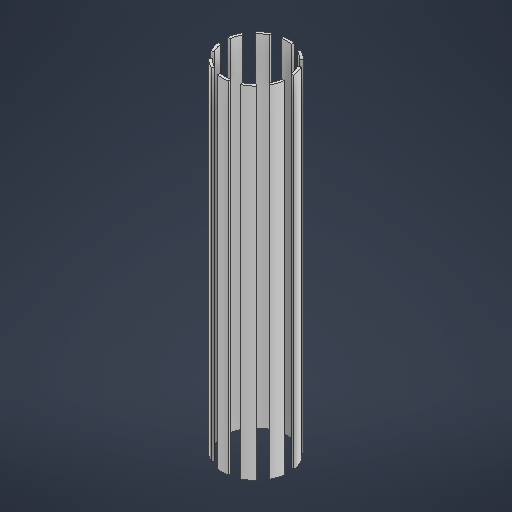
# Autodesk Inventor part: bandstoproller
Saved by Autodesk Inventor 2026.1 (Build 301233000, 233)
## iProperties
Created: 2025-08-08
Part Number: bandstoproller
Material: Generic
Document SubType Name: Modeling
Designer: roejo
Density: 1 g/cm^3
Appearance: Default
Author: roejo
Autodesk Inventor part; units mm, degrees
ref_plane "YZ Plane" through (0, 0, 0) normal (1, 0, 0) x (0, 1, 0)
ref_plane "XZ Plane" through (0, 0, 0) normal (0, 1, 0) x (-1, 0, 0)
ref_plane "XY Plane" through (0, 0, 0) normal (0, 0, 1) x (1, 0, 0)
sketch "Sketch1" plane through (0, 0, 0) normal (0, 1, 0) x (-1, 0, 0)
  circle A0 centre (0, 0) radius 20.6375
  dimension "d0" = 41.275
  constraints: 1 centre point, 1 coincident
  measures "d0" diameter of A0
extrude "Extrusion1" add sketch "Sketch1" along normal blind 211.0232
sketch "Sketch2" plane through (0, 211.0232, 0) normal (0, 1, 0) x (1, 0, 0)
  circle A0 centre (0, 0) radius 19.05
  dimension "d3" = 38.1
  constraints: 1 centre point, 1 coincident
  measures "d3" diameter of A0
extrude "Extrusion2" cut sketch "Sketch2" against normal through all
sketch "Sketch3" plane through (0, 211.0232, 0) normal (0, 1, 0) x (1, 0, 0)
  line L0 (-25.4, -2.8575) -> (-12.7, -2.8575)
  line L1 (-12.7, -2.8575) -> (-12.7, 2.8575)
  line L2 (-12.7, 2.8575) -> (-25.4, 2.8575)
  line L3 (-25.4, 2.8575) -> (-25.4, -2.8575)
  line L4 (-18.8694, -17.2415) -> (-8.5949, -9.7766)
  line L5 (-8.5949, -9.7766) -> (-11.9541, -5.1531)
  line L6 (-11.9541, -5.1531) -> (-22.2286, -12.618)
  line L7 (-22.2286, -12.618) -> (-18.8694, -17.2415)
  line L8 (-5.1314, -25.0399) -> (-1.2069, -12.9614)
  line L9 (-1.2069, -12.9614) -> (-6.6422, -11.1954)
  line L10 (-6.6422, -11.1954) -> (-10.5667, -23.2738)
  line L11 (-10.5667, -23.2738) -> (-5.1314, -25.0399)
  line L12 (10.5667, -23.2738) -> (6.6422, -11.1954)
  line L13 (6.6422, -11.1954) -> (1.2069, -12.9614)
  line L14 (1.2069, -12.9614) -> (5.1314, -25.0399)
  line L15 (5.1314, -25.0399) -> (10.5667, -23.2738)
  line L16 (22.2286, -12.618) -> (11.9541, -5.1531)
  line L17 (11.9541, -5.1531) -> (8.5949, -9.7766)
  line L18 (8.5949, -9.7766) -> (18.8694, -17.2415)
  line L19 (18.8694, -17.2415) -> (22.2286, -12.618)
  line L20 (25.4, 2.8575) -> (12.7, 2.8575)
  line L21 (12.7, 2.8575) -> (12.7, -2.8575)
  line L22 (12.7, -2.8575) -> (25.4, -2.8575)
  line L23 (25.4, -2.8575) -> (25.4, 2.8575)
  line L24 (18.8694, 17.2415) -> (8.5949, 9.7766)
  line L25 (8.5949, 9.7766) -> (11.9541, 5.1531)
  line L26 (11.9541, 5.1531) -> (22.2286, 12.618)
  line L27 (22.2286, 12.618) -> (18.8694, 17.2415)
  line L28 (5.1314, 25.0399) -> (1.2069, 12.9614)
  line L29 (1.2069, 12.9614) -> (6.6422, 11.1954)
  line L30 (6.6422, 11.1954) -> (10.5667, 23.2738)
  line L31 (10.5667, 23.2738) -> (5.1314, 25.0399)
  circle A0 centre (0, 0) radius 20.6375 projected
  line L32 (-10.5667, 23.2738) -> (-6.6422, 11.1954)
  line L33 (-6.6422, 11.1954) -> (-1.2069, 12.9614)
  line L34 (-1.2069, 12.9614) -> (-5.1314, 25.0399)
  line L35 (-5.1314, 25.0399) -> (-10.5667, 23.2738)
  line L36 (-22.2286, 12.618) -> (-11.9541, 5.1531)
  line L37 (-11.9541, 5.1531) -> (-8.5949, 9.7766)
  line L38 (-8.5949, 9.7766) -> (-18.8694, 17.2415)
  line L39 (-18.8694, 17.2415) -> (-22.2286, 12.618)
  point P0 (-30.1625, 0)
  point P1 (-24.402, -17.7291)
  point P2 (-9.3207, -28.6862)
  point P3 (9.3207, -28.6862)
  point P4 (24.402, -17.7291)
  point P5 (30.1625, 0)
  point P6 (24.402, 17.7291)
  point P7 (9.3207, 28.6862)
  point P8 (-9.3207, 28.6862)
  point P9 (-24.402, 17.7291)
  dimension "d13" = 360
  dimension "d16" = 12.7
  constraints: 80 end point, 2 parallel, 1 horizontal, 1 perpendicular, 91 other
  measures "d16" distance from line of A0.centre L1
extrude "Extrusion3" cut sketch "Sketch3" against normal through all contours L3 L2 A0 L0 | A0 L2 L1 L0 | A0 L4 L7 L6 | L6 L5 L4 A0 | L36 L39 L38 A0 | A0 L38 L37 L36 | A0 L8 L11 L10 | L10 L9 L8 A0 | L32 L35 L34 A0 | A0 L34 L33 L32 | A0 L12 L15 L14 | L14 L13 L12 A0 | A0 L30 L29 L28 | L28 L31 L30 A0 | A0 L16 L19 L18 | L18 L17 L16 A0 | A0 L26 L25 L24 | L24 L27 L26 A0 | A0 L20 L23 L22 | L22 L21 L20 A0
body "Solid1"
